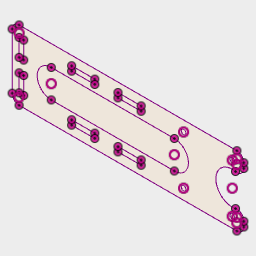
assembled (Autodesk Fusion 360 archive; units mm, degrees)
design "Lower Leg"
Autodesk Fusion 360 part; units mm, degrees
sketch "Sketch1" plane through (0, 0, -20.5) normal (0, 0, -1) x (-1, 0, 0)
  line L0 (-5, 0) -> (-5, -15)
  line L1 (-5, -15) -> (95, -15)
  line L2 (95, -15) -> (95, 0)
  circle A0 centre (0, -10.5) radius 1
  circle A1 centre (21, -10.5) radius 1
  circle A2 centre (0, 0) radius 7.0711
  line L3 (92, -10.3624) -> (90, -10.3624)
  line L4 (90, -10.3624) -> (90, -2.8871)
  line L5 (90, -2.8871) -> (92, -2.8871)
  line L6 (92, -2.8871) -> (92, -10.3624)
  line L7 (100, 0) -> (42, 0) construction
  line L8 (-5, 15) -> (95, 15)
  line L9 (95, 15) -> (95, 0)
  line L10 (92, 10.3624) -> (90, 10.3624)
  line L11 (92, 2.8871) -> (92, 10.3624)
  line L12 (90, 10.3624) -> (90, 2.8871)
  line L13 (90, 2.8871) -> (92, 2.8871)
  circle A3 centre (21, 10.5) radius 1
  circle A4 centre (0, 10.5) radius 1
  line L14 (-5, 0) -> (-5, 15)
  line L15 (39.3215, 11.0949) -> (49.3215, 11.0949)
  line L16 (49.3215, 11.0949) -> (49.3215, 9.0949)
  line L17 (49.3215, 9.0949) -> (39.3215, 9.0949)
  line L18 (39.3215, 9.0949) -> (39.3215, 11.0949)
  line L19 (54.3215, 11.5) -> (54.3215, -12) construction
  line L20 (54.3215, -11.5) -> (54.3215, 12) construction
  line L21 (49.3215, -11.0949) -> (49.3215, -9.0949)
  line L22 (49.3215, -9.0949) -> (39.3215, -9.0949)
  line L23 (39.3215, -9.0949) -> (39.3215, -11.0949)
  line L24 (39.3215, -11.0949) -> (49.3215, -11.0949)
  line L25 (69.3215, 11.0949) -> (59.3215, 11.0949)
  line L26 (59.3215, 11.0949) -> (59.3215, 9.0949)
  line L27 (59.3215, 9.0949) -> (69.3215, 9.0949)
  line L28 (69.3215, 9.0949) -> (69.3215, 11.0949)
  line L29 (59.3215, -11.0949) -> (59.3215, -9.0949)
  line L30 (69.3215, -9.0949) -> (69.3215, -11.0949)
  line L31 (59.3215, -9.0949) -> (69.3215, -9.0949)
  line L32 (69.3215, -11.0949) -> (59.3215, -11.0949)
  dimension "d1" = 100
  dimension "d3" = 2
  dimension "d4" = 3
  dimension "d77" = 0
  dimension "d78" = 0
  dimension "d79" = 0
  dimension "d80" = 0
  dimension "d93" = 10
  dimension "d94" = 2
  dimension "d95" = 10
  measures "d1" distance of L0.end L1.end
  measures "d3" distance of L4 L6
  measures "d4" distance of L2 L6
  measures "d93" distance of L15.start L15.end
  measures "d94" distance of L15.start L17.end
  measures "d95" distance of L16 L26
extrude "Extrude1" add sketch "Sketch1" along normal blind 2 contours L0 L1 L2 A2 L8 L9 L14
sketch "Sketch2" plane through (0, 0, -22.5) normal (0, 0, -1) x (-1, 0, 0)
  line L0 (25, -6.0704) -> (78.1149, -6.0704)
  arc A0 (78.1149, -6.0704) -> (78.1149, 6.0704) centre (78.1149, 0) ccw
  line L1 (78.1149, 6.0704) -> (25, 6.0704)
  arc A1 (25, 6.0704) -> (25, -6.0704) centre (25, 0) ccw
  line L2 (25, 0) -> (78.1149, 0) construction
extrude "Extrude2" cut sketch "Sketch2" against normal blind 2
fillet "Fillet1" radius 3 6 edges at (5, 15, -21.5) (5, 5, -21.5) (5, -5, -21.5) (5, -15, -21.5) (-95, 15, -21.5) (-95, -15, -21.5)
sketch "Sketch3" plane through (0, 0, -20.5) normal (0, 0, 1) x (1, 0, 0)
sketch "Projection" plane through (0, 0, -20.5) normal (0, 0, 1) x (1, 0, 0)
  line L0 (-25, -6.0704) -> (-78.1149, -6.0704)
  arc A0 (-78.1149, 6.0704) -> (-78.1149, -6.0704) centre (-78.1149, 0) ccw
  line L1 (-78.1149, 6.0704) -> (-25, 6.0704)
  arc A1 (-25, -6.0704) -> (-25, 6.0704) centre (-25, 0) ccw
  line L2 (-92, -2.8871) -> (-90, -2.8871)
  line L3 (-90, -2.8871) -> (-90, -10.3624)
  line L4 (-90, -10.3624) -> (-92, -10.3624)
  line L5 (-92, -10.3624) -> (-92, -2.8871)
  line L6 (-39.3215, -11.0949) -> (-49.3215, -11.0949)
  line L7 (-49.3215, -11.0949) -> (-49.3215, -9.0949)
  line L8 (-49.3215, -9.0949) -> (-39.3215, -9.0949)
  line L9 (-39.3215, -9.0949) -> (-39.3215, -11.0949)
  line L10 (-69.3215, 9.0949) -> (-69.3215, 11.0949)
  line L11 (-69.3215, 11.0949) -> (-59.3215, 11.0949)
  line L12 (-59.3215, 11.0949) -> (-59.3215, 9.0949)
  line L13 (-59.3215, 9.0949) -> (-69.3215, 9.0949)
  circle A2 centre (-21, -10.5) radius 1
  circle A3 centre (-21, 10.5) radius 1
  line L14 (-69.3215, -11.0949) -> (-69.3215, -9.0949)
  line L15 (-69.3215, -9.0949) -> (-59.3215, -9.0949)
  line L16 (-59.3215, -9.0949) -> (-59.3215, -11.0949)
  line L17 (-59.3215, -11.0949) -> (-69.3215, -11.0949)
  line L18 (-90, 2.8871) -> (-92, 2.8871)
  line L19 (-92, 2.8871) -> (-92, 10.3624)
  line L20 (-92, 10.3624) -> (-90, 10.3624)
  line L21 (-90, 10.3624) -> (-90, 2.8871)
  circle A4 centre (0, 10.5) radius 1
  line L22 (-39.3215, 9.0949) -> (-49.3215, 9.0949)
  line L23 (-49.3215, 9.0949) -> (-49.3215, 11.0949)
  line L24 (-49.3215, 11.0949) -> (-39.3215, 11.0949)
  line L25 (-39.3215, 11.0949) -> (-39.3215, 9.0949)
  circle A5 centre (0, -10.5) radius 1
  arc A6 (-95, -12) -> (-92, -15) centre (-92, -12) ccw
  line L26 (-92, -15) -> (2, -15)
  arc A7 (2, -15) -> (5, -12) centre (2, -12) ccw
  line L27 (5, -12) -> (5, -9.8705)
  arc A8 (5, -9.8705) -> (1.4042, -6.9302) centre (2, -9.8705) ccw
  arc A9 (1.4042, 6.9302) -> (1.4042, -6.9302) centre (0, 0) ccw
  arc A10 (1.4042, 6.9302) -> (5, 9.8705) centre (2, 9.8705) ccw
  line L28 (5, 9.8705) -> (5, 12)
  arc A11 (5, 12) -> (2, 15) centre (2, 12) ccw
  line L29 (2, 15) -> (-92, 15)
  arc A12 (-92, 15) -> (-95, 12) centre (-92, 12) ccw
  line L30 (-95, 12) -> (-95, -12)
equation "thiccness = 2 mm"
equation "d3 = thiccness"
equation "d11 = thiccness"
equation "d94 = thiccness"
equation "d96 = -thiccness"
named bodies: "leg"
